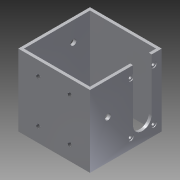
# Autodesk Inventor part: 04
Saved by Autodesk Inventor 2013 (Build 170138000, 138)
## iProperties
Created: 2014-02-01
Material: アルミニウム 6061
Document SubType Name: Modeling
Designer: andou
Density: 2.71 g/cm^3
Mass: 48.6262 g
Surface Area: 190.981 cm^2
Volume: 17.9432 cm^3
Part Number: 04
Author: andou
Title: Left_Parallel_Case
Autodesk Inventor part; units mm, degrees
ref_plane "YZ Plane" through (0, 0, 0) normal (1, 0, 0) x (0, 1, 0)
ref_plane "XZ Plane" through (0, 0, 0) normal (0, 1, 0) x (-1, 0, 0)
ref_plane "XY Plane" through (0, 0, 0) normal (0, 0, 1) x (1, 0, 0)
sketch "スケッチ1" plane through (0, 0, 0) normal (0, 0, 1) x (1, 0, 0)
  line L0 (-25, 25) -> (25, 25)
  line L1 (25, 25) -> (25, -25)
  line L2 (25, -25) -> (-25, -25)
  line L3 (-25, -25) -> (-25, 25)
  line L4 (-23, 23) -> (23, 23)
  line L5 (23, 23) -> (23, -23)
  line L6 (23, -23) -> (-23, -23)
  line L7 (-23, -23) -> (-23, 23)
  point P0 (0, 0)
  dimension "d0" = 50
  dimension "d1" = 50
  dimension "d4" = 25
  dimension "d5" = 25
  dimension "d6" = 46
  dimension "d7" = 2
  dimension "d8" = 46
  dimension "d9" = 2
  constraints: 16 end point, 4 parallel, 2 horizontal, 2 perpendicular
  measures "d0" distance of L0.start L0.end
  measures "d1" distance of L2.end L0.start
  measures "d4" distance from line of L0 point (0, 0)
  measures "d5" distance from line of L3 point (0, 0)
  measures "d6" distance between parallel lines of L5 L7
  measures "d7" distance between parallel lines of L3 L7
  measures "d8" distance between parallel lines of L4 L6
  measures "d9" distance between parallel lines of L2 L6
extrude "押し出し1" add sketch "スケッチ1" along normal blind 50
sketch "スケッチ2" plane through (25, -25, 0) normal (1, 0, 0) x (0, 0, -1)
  line L0 (-50, 50) -> (-50, 0) projected
  line L1 (-50, 43) -> (-13.5, 43)
  line L2 (-13.5, 30) -> (-50, 30)
  line L3 (-50, 30) -> (-50, 43)
  arc A0 (-13.5, 30) -> (-13.5, 43) centre (-13.5, 36.5) ccw
  line L4 (0, 50) -> (-50, 50) projected
  point P0 (0, 25)
  point P1 (-11.7323, 30.245)
  dimension "d34" = 13
  dimension "d43" = 13
  dimension "d44" = 6.5
  dimension "d46" = 36.5
  dimension "d236" = 7
  constraints: 6 end point, 3 point on circle, 1 centre point, 1 horizontal, 1 parallel, 1 point on line
  measures "d34" distance between parallel lines of L1 L2
  measures "d43" diameter of A0
  measures "d44" distance from line of L2 A0.centre
  measures "d46" distance from line of L0 A0.centre
  measures "d236" distance between parallel lines of L4 L1
extrude "押し出し2" cut sketch "スケッチ2" against normal blind 30.5
sketch "スケッチ3" plane through (25, -25, 0) normal (1, 0, 0) x (0, 0, -1)
  arc A0 (-13.5, 30) -> (-13.5, 43) centre (-13.5, 36.5) ccw projected
  line L0 (-13.5, 30) -> (-50, 30) projected
  circle A1 centre (-7, 44.5) radius 1
  circle A2 centre (-43, 44.5) radius 1
  circle A3 centre (-43, 28.5) radius 1
  circle A4 centre (-7, 28.5) radius 1
  point P0 (0, 25)
  dimension "d47" = 8
  dimension "d48" = 8
  dimension "d49" = 16
  dimension "d50" = 1.5
  dimension "d51" = 36
  dimension "d52" = 36
  dimension "d53" = 6.5
  dimension "d55" = 2
  dimension "d56" = 6.5
  constraints: 4 centre point, 3 equal radius
  measures "d47" vertical distance of A1.centre A0.centre
  measures "d48" vertical distance of A0.centre A4.centre
  measures "d49" distance of A2.centre A3.centre
  measures "d50" distance from line of L0 A3.centre
  measures "d51" distance of A1.centre A2.centre
  measures "d52" distance of A4.centre A3.centre
  measures "d53" horizontal distance of A0.centre A4.centre
  measures "d55" diameter of A4
  measures "d56" horizontal distance of A0.centre A1.centre
hole "穴1" at (25, 3.5, 43) at (25, 19.5, 7) at (25, 3.5, 7) at (25, 19.5, 43) direction (-1, 0, 0) diameter 2 depth 2 tip angle 118 counterbore diameter 4 counterbore depth 0.5
sketch "スケッチ11" plane through (25, -25, 0) normal (1, 0, 0) x (0, 0, -1)
  circle A0 centre (-36.5, 36.5) radius 1.5
  line L0 (-50, 50) -> (-50, 43) projected
  circle A1 centre (-27.5, 12.5) radius 1.5
  line L1 (0, 50) -> (0, 0) projected
  line L2 (0, 50) -> (-50, 50) projected
  point P0 (0, 25)
  dimension "d109" = 3
  dimension "d128" = 24
  dimension "d237" = 13.5
  dimension "d238" = 27.5
  dimension "d239" = 13.5
  constraints: 2 centre point, 1 equal radius
  measures "d109" diameter of A0
  measures "d128" vertical distance of A1.centre A0.centre
  measures "d237" distance from line of L2 A0.centre
  measures "d238" distance from line of L1 A1.centre
  measures "d239" distance from line of L0 A0.centre
hole "穴6" at (25, -12.5, 27.5) at (25, 11.5, 36.5) direction (-1, 0, 0) diameter 4 end through all
sketch "スケッチ18" plane through (-25, -25, 0) normal (0, -1, 0) x (1, 0, 0)
  line L0 (50, 50) -> (0, 50) projected
  line L1 (50, 0) -> (0, 0) projected
  circle A0 centre (14, 40) radius 1.5
  circle A1 centre (36, 40) radius 1.5
  circle A2 centre (14, 10) radius 1.5
  circle A3 centre (36, 10) radius 1.5
  line L2 (0, 0) -> (0, 50) projected
  line L3 (50, 0) -> (50, 50) projected
  point P0 (49.5, 0)
  point P1 (49.5, 50)
  point P2 (25, 0)
  dimension "d240" = 10
  dimension "d241" = 10
  dimension "d242" = 10
  dimension "d243" = 10
  dimension "d248" = 3
  dimension "d267" = 22
  dimension "d268" = 22
  dimension "d269" = 14
  dimension "d270" = 14
  constraints: 4 centre point, 3 equal radius
  measures "d240" distance from line of L1 A2.centre
  measures "d241" distance from line of L1 A3.centre
  measures "d242" distance from line of L0 A0.centre
  measures "d243" distance from line of L0 A1.centre
  measures "d248" diameter of A3
  measures "d267" distance of A1.centre A0.centre
  measures "d268" distance of A3.centre A2.centre
  measures "d269" distance from line of L3 A3.centre
  measures "d270" distance from line of L2 A0.centre
hole "穴13" at (-11, -25, 40) at (-11, -25, 10) at (11, -25, 40) at (11, -25, 10) direction (0, 1, 0) diameter 3 depth 2 tip angle 118
thread "ねじ13" size "M3x0.5" class "6H" standard "ANSI Metric M Profile" full length
thread "ねじ14" size "M3x0.5" class "6H" standard "ANSI Metric M Profile" full length
thread "ねじ15" size "M3x0.5" class "6H" standard "ANSI Metric M Profile" full length
thread "ねじ16" size "M3x0.5" class "6H" standard "ANSI Metric M Profile" full length
